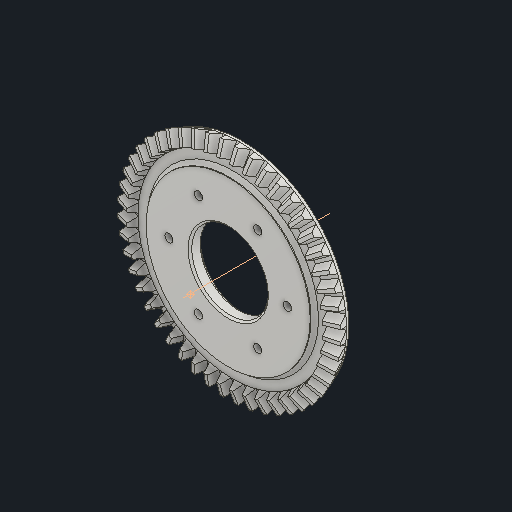
# Autodesk Inventor part: ENGRANAJE CÓNICO 1
Saved by Autodesk Inventor 2022 (Build 260153000, 153)
## iProperties
CustomPartVersion: 1
Created: 2021-09-21
Part Number: ENGRANAJE CÓNICO 1
Material: Steel, Mild
Document SubType Name: Modeling
Designer: Andres
Categories: <?xml version="1.0" encoding="UTF-16"?> <MemberInstance><Categories><FamilyTemplate><FamilyTemplateParameter ValueType="xs:double" Id="1" ObjectReferenceKey="da_z" ObjectType="kUserParameterObject"/><FamilyTemplateParameter ValueType="xs:double" Id="2" ObjectReferenceKey="da_b" ObjectType="kUserParameterObject"/><FamilyTemplateParameter ValueType="xs:double" Id="3" ObjectReferenceKey="da_beta" ObjectType="kUserParameterObject"/><FamilyTemplateParameter ValueType="xs:double" Id="4" ObjectReferenceKey="da_dae" ObjectType="kUserParameterObject"/><FamilyTemplateParameter ValueType="xs:double" Id="5" ObjectReferenceKey="da_ve" ObjectType="kUserParameterObject"/><FamilyTemplateParameter ValueType="xs:double" Id="6" ObjectReferenceKey="da_omega" ObjectType="kUserParameterObject"/><FamilyTemplateParameter ValueType="xs:string" Id="7" ObjectReferenceKey="EAIAABAAAAAAHwAAAAAAAIAAAAAAAAAA" ObjectType="83914240" SubObjectId="SurfaceGeometry"/></FamilyTemplate><ParamToTemplateMap><ParamToTemplate CategoryParameter="//CategoryParameter[@InternalName='046C89C9-8512-4d59-83FE-43B91F4F132A']" TemplateParameter="1"/><ParamToTemplate CategoryParameter="//CategoryParameter[@InternalName='2552DF32-E462-4b46-AEBF-C6C7768E72AC']" TemplateParameter="2"/><ParamToTemplate CategoryParameter="//CategoryParameter[@InternalName='C9EE641D-15FC-4fae-A226-E94C4372FDD7']" TemplateParameter="3"/><ParamToTemplate><ParamToTemplate CategoryParameter="//CategoryParameter[@InternalName='00B6519A-459B-49c7-AD84-2E56D39A5744']" ConstantValue="0.378492"/></ParamToTemplate><ParamToTemplate><ParamToTemplate CategoryParameter="//CategoryParameter[@InternalName='04B31F0E-C7A6-4894-AA32-9629BEFACF47']" ConstantValue="1.000000"/></ParamToTemplate><ParamToTemplate><ParamToTemplate CategoryParameter="//CategoryParameter[@InternalName='43CBEC2E-7847-49e7-A936-2F7889FCB2D9']" ConstantValue="0.200000"/></ParamToTemplate><ParamToTemplate><ParamToTemplate CategoryParameter="//CategoryParameter[@InternalName='B1EFC894-105D-4ebd-86BF-FA20ED196853']" ConstantValue="0.300000"/></ParamToTemplate><ParamToTemplate><ParamToTemplate CategoryParameter="//CategoryParameter[@InternalName='51175063-3D10-4879-93E8-6246FE8B403D']" ConstantValue="2060000000.000000"/></ParamToTemplate><ParamToTemplate><ParamToTemplate CategoryParameter="//CategoryParameter[@InternalName='A3A52E27-4454-46a9-B0BD-C932399B70AF']" ConstantValue="0.300000"/></ParamToTemplate><ParamToTemplate CategoryParameter="//CategoryParameter[@InternalName='2A200944-5A8C-41ca-B96E-8520D2E510F1']" TemplateParameter="4"/><ParamToTemplate><ParamToTemplate CategoryParameter="//CategoryParameter[@InternalName='1A637F62-92C8-44bc-B81F-10802510B579']" ConstantValue="10.734536"/></ParamToTemplate><ParamToTemplate CategoryParameter="//CategoryParameter[@InternalName='B52DD4BE-6863-48fb-BF58-89EF6F9EC65C']" TemplateParameter="5"/><ParamToTemplate><ParamToTemplate CategoryParameter="//CategoryParameter[@InternalName='3956BFF2-84D2-457d-93C2-9B0613DEBA67']" ConstantValue="1.799854"/></ParamToTemplate><ParamToTemplate CategoryParameter="//CategoryParameter[@InternalName='739CFA02-461B-4bf8-8049-181FCAD8B28F']" TemplateParameter="6"/><ParamToTemplate><ParamToTemplate CategoryParameter="//CategoryParameter[@InternalName='A27E999F-E2CE-4481-8A2A-EBF499C4C3C5']" ConstantValue="0.000000"/></ParamToTemplate><ParamToTemplate><ParamToTemplate CategoryParameter="//CategoryParameter[@InternalName='9E1B4470-B2D3-4ff1-B813-535BB4CDF51A']" ConstantValue="3160000.000000"/></ParamToTemplate><ParamToTemplate><ParamToTemplate CategoryParameter="//CategoryParameter[@InternalName='F8452263-BFF6-458c-9FB1-07C4B99E95CD']" ConstantValue="11400000.000000"/></ParamToTemplate><ParamToTemplate><ParamToTemplate CategoryParameter="//CategoryParameter[@InternalName='3E3BB259-FD49-497f-8171-6EBC954A3479']" ConstantValue="2.000000"/></ParamToTemplate><ParamToTemplate CategoryParameter="//CategoryParameter[@InternalName='27C3BAF2-7550-4e4b-AE2C-0DB134B7D9B7']" TemplateParameter="7"/></ParamToTemplateMap><Category DisplayName="Gear" InternalName="DC85795E-93AB-48d5-8EEE-5A27447B64BD" Mnemonic="Gear"><CategoryParameter DisplayName="z" InternalName="046C89C9-8512-4d59-83FE-43B91F4F132A" Mnemonic="z"/><CategoryParameter DisplayName="b" InternalName="2552DF32-E462-4b46-AEBF-C6C7768E72AC" Mnemonic="b"/><CategoryParameter DisplayName="||b|" InternalName="C9EE641D-15FC-4fae-A226-E94C4372FDD7" Mnemonic="beta"/><CategoryParameter DisplayName="x" InternalName="00B6519A-459B-49c7-AD84-2E56D39A5744" Mnemonic="x"/><CategoryParameter DisplayName="a*" InternalName="04B31F0E-C7A6-4894-AA32-9629BEFACF47" Mnemonic="a"/><CategoryParameter DisplayName="c*" InternalName="43CBEC2E-7847-49e7-A936-2F7889FCB2D9" Mnemonic="c"/><CategoryParameter DisplayName="r|.f|*" InternalName="B1EFC894-105D-4ebd-86BF-FA20ED196853" Mnemonic="rf"/><CategoryParameter DisplayName="E" InternalName="51175063-3D10-4879-93E8-6246FE8B403D" Mnemonic="E"/><CategoryParameter DisplayName="||m|" InternalName="A3A52E27-4454-46a9-B0BD-C932399B70AF" Mnemonic="mi"/><Category DisplayName="BevelGear" InternalName="0C98F69A-0C2B-4791-B2FE-7691BB227E77" Mnemonic="BevelGear"><CategoryParameter DisplayName="d|.ae|" InternalName="2A200944-5A8C-41ca-B96E-8520D2E510F1" Mnemonic="dae"/><CategoryParameter DisplayName="d|.ai|" InternalName="1A637F62-92C8-44bc-B81F-10802510B579" Mnemonic="dai"/><CategoryParameter DisplayName="A|.e|" InternalName="B52DD4BE-6863-48fb-BF58-89EF6F9EC65C" Mnemonic="ve"/><CategoryParameter DisplayName="A|.i|" InternalName="3956BFF2-84D2-457d-93C2-9B0613DEBA67" Mnemonic="vi"/><CategoryParameter DisplayName="||S|" InternalName="739CFA02-461B-4bf8-8049-181FCAD8B28F" Mnemonic="omega"/><CategoryParameter DisplayName="x|.t|" InternalName="A27E999F-E2CE-4481-8A2A-EBF499C4C3C5" Mnemonic="xt"/><CategoryParameter DisplayName="||s||.Flim|" InternalName="9E1B4470-B2D3-4ff1-B813-535BB4CDF51A" Mnemonic="sFlim"/><CategoryParameter DisplayName="||s||.Hlim|" InternalName="F8452263-BFF6-458c-9FB1-07C4B99E95CD" Mnemonic="sHlim"/><CategoryParameter DisplayName="type" InternalName="3E3BB259-FD49-497f-8171-6EBC954A3479" Mnemonic="type"/><CategoryParameter DisplayName="PitchDiameter" InternalName="27C3BAF2-7550-4e4b-AE2C-0DB134B7D9B7" Mnemonic="IDS_PITCHDIAM"/></Category></Category></Categories></MemberInstance>
Mass: 60.9118 g
Surface Area: 34.3074 cm^2
Volume: 7.7496 cm^3
Density: 7.86 g/cm^3
Appearance: Steel
Author: Andres
Autodesk Inventor part; units mm, degrees
ref_plane "Mesh Plane2" through (0, 0, 0) normal (0.9978589, 0.0654031, 0) x (0, 0, 1)
sketch "Teeth Body Sketch" plane through (0, 0, 0) normal (1, 0, 0) x (0, 1, 0)
  line L0 (0, 0) -> (59.2441, -25.6596) construction
  line L1 (59.2441, -25.6596) -> (61.2684, -20.5457)
  line L2 (61.2684, -20.5457) -> (0, 0) construction
  line L3 (60, -23.75) -> (0, 0) construction
  line L4 (51.8994, -22.4785) -> (53.6727, -17.9985)
  line L5 (59.2441, -25.6596) -> (51.8994, -22.4785)
  line L6 (61.2684, -20.5457) -> (53.6727, -17.9985)
  line L7 (0, -30.7915) -> (0, 5.1319) projected
  line L8 (0, -23.75) -> (61.2684, -23.75) construction
  dimension "d0" = 120
  dimension "d1" = 118.4882
  dimension "d2" = 122.5368
  dimension "d3" = 8
  dimension "d4" = 20.5457
  constraints: 16 end point, 4 point on line, 3 perpendicular, 2 collinear, 1 horizontal alignment, 1 vertical alignment
  measures "d0" diameter of L3.start L7
  measures "d1" diameter of L0.end L7
  measures "d2" diameter of L1.end L7
  measures "d3" distance between parallel lines of L1 L4
  measures "d4" vertical distance of L1.end L0.start
revolve "Teeth Body" add sketch "Teeth Body Sketch" angle 360 about axis through (0, 0, 0) along (0, 0, 1)
ref_plane "Tooth Plane" through (0, 60, -23.75) normal (0, -0.9298066, 0.3680485) x (1, 0, 0)
sketch "Start Sketch" plane through (0, 60, -23.75) normal (0, -0.9298066, 0.3680485) x (1, 0, 0)
  line L0 (0, -196.6479) -> (0, 38.7332) projected
  arc A0 (-0.741, -2.7138) -> (-3.7477, 5.0545) centre (-57.4116, -20.1822) ccw
  arc A1 (3.7477, 5.0545) -> (0.741, -2.7138) centre (57.4116, -20.1822) ccw
  line L1 (-0.741, -2.7138) -> (0.741, -2.7138)
  arc A2 (3.7477, 5.0545) -> (-3.7477, 5.0545) centre (0, -163.022) ccw
  dimension "d7" = 59.3018
  dimension "d8" = 57.4116
  dimension "d9" = 142.8398
  dimension "d57" = 168.1182
  dimension "d58" = 160.3082
  constraints: 6 point on circle, 3 centre point, 3 symmetric about line, 2 end point, 1 coincident, 1 perpendicular, 1 other
  measures "d7" radius of A0
  measures "d8" horizontal distance of point (0, -163.022) A0.centre
  measures "d9" vertical distance of point (0, -163.022) A0.centre
  measures "d57" radius of A2
  measures "d58" distance from line of A2.centre L1
sketch "End Sketch" plane through (0, 52.3059, -20.7044) normal (0, -0.9298066, 0.3680485) x (1, 0, 0)
  line L0 (0, -171.4306) -> (0, 33.7662) projected
  arc A0 (-0.646, -2.3658) -> (-3.2671, 4.4063) centre (-50.0494, -17.5941) ccw
  arc A1 (3.2671, 4.4063) -> (0.646, -2.3658) centre (50.0494, -17.5941) ccw
  line L1 (-0.646, -2.3658) -> (0.646, -2.3658)
  arc A2 (3.2671, 4.4063) -> (-3.2671, 4.4063) centre (0, -142.1168) ccw
  dimension "d12" = 51.6972
  dimension "d15" = 50.0494
  dimension "d16" = 124.5226
  dimension "d59" = 146.5595
  dimension "d60" = 139.751
  constraints: 6 point on circle, 3 centre point, 3 symmetric about line, 2 end point, 1 coincident, 1 other
  measures "d12" radius of A0
  measures "d15" horizontal distance of A0.centre point (0, -142.117)
  measures "d16" vertical distance of A0.centre point (0, -142.117)
  measures "d59" radius of A2
  measures "d60" distance from line of A2.centre L1
loft "Loft" cut profiles "Start Sketch", "End Sketch"
pattern_circular "Circular Pattern" count 48 over 360 about axis through (0, 0, 0) along (0, 0, 1) of "Loft"
ref_plane "End Plane" through (0, 52.3059, -20.7044) normal (0, -0.9298066, 0.3680485) x (1, 0, 0)
sketch3d "3D Sketch Right"
ref_plane "End Plane Right" through (-2.7978, 52.231, -20.7044) normal (0.0497347, -0.9284755, 0.3680485) x (0.9985684, 0.0534892, 0)
sketch "End Sketch Right" plane through (-2.7978, 52.231, -20.7044) normal (0.0497347, -0.9284755, 0.3680485) x (0.9985684, 0.0534892, 0)
  arc A0 (-0.646, -2.3658) -> (-3.2671, 4.4063) centre (-50.0494, -17.5941) ccw
  line L0 (0, -174.1855) -> (0, 36.5211) projected
  arc A1 (3.2671, 4.4063) -> (0.646, -2.3658) centre (50.0494, -17.5941) ccw
  line L1 (-0.646, -2.3658) -> (0.646, -2.3658)
  arc A2 (3.2671, 4.4063) -> (-3.2671, 4.4063) centre (0, -142.1168) ccw
  dimension "d70" = 50.0494
  dimension "d71" = 124.5226
  dimension "d72" = 51.6972
  dimension "d73" = 139.751
  dimension "d74" = 146.5595
  constraints: 6 point on circle, 3 centre point, 3 symmetric about line, 2 end point, 1 coincident, 1 perpendicular, 1 other
  measures "d70" horizontal distance of A2.centre A0.centre
  measures "d71" vertical distance of point (0, -142.117) A0.centre
  measures "d72" radius of A0
  measures "d73" distance from line of point (0, -142.117) L1
  measures "d74" radius of A2
feature "Loft Right" [suppressed]
pattern_circular "Circular Pattern Right" [suppressed]
sketch3d "3D Sketch Left"
ref_plane "End Plane Left" through (2.8193, 52.231, -20.7243) normal (-0.0501091, -0.928337, 0.3683469) x (0.9985464, -0.0538988, 0)
sketch "End Sketch Left" plane through (2.8193, 52.231, -20.7243) normal (-0.0501091, -0.928337, 0.3683469) x (0.9985464, -0.0538988, 0)
  line L0 (0, -174.3918) -> (0, 36.7636) projected
  arc A0 (-0.646, -2.3477) -> (-3.2671, 4.4244) centre (-50.0494, -17.576) ccw
  arc A1 (3.2671, 4.4244) -> (0.646, -2.3477) centre (50.0494, -17.576) ccw
  line L1 (-0.646, -2.3477) -> (0.646, -2.3477)
  ellipse E0 centre (0, -16.733) end of major axis (53.6727, -16.733) minor radius 19.7702 projected
  arc A2 (3.2671, 4.4244) -> (-3.2671, 4.4244) centre (0, -142.0987) ccw
  point P0 (0, -142.0987)
  dimension "d56" = 19.7702
  dimension "d30" = 51.6972
  dimension "d31" = 50.0494
  dimension "d32" = 124.5226
  dimension "d61" = 146.5595
  dimension "d62" = 139.751
  constraints: 6 point on circle, 3 centre point, 3 symmetric about line, 2 end point, 1 coincident, 2 other
  measures "d30" radius of A0
  measures "d31" horizontal distance of point (0, -142.099) A0.centre
  measures "d32" vertical distance of A0.centre point (0, -142.099)
  measures "d61" radius of A2
  measures "d62" distance from line of point (0, -142.099) L1
feature "Loft Left" [suppressed]
pattern_circular "Circular Pattern Left" [suppressed]
sketch "Body Sketch" plane through (0, 0, 0) normal (1, 0, 0) x (0, 1, 0)
  line L0 (0, -26.2958) -> (0, -21.8423) projected
  line L1 (59.2441, -25.6596) -> (51.8994, -22.4785) projected
  line L2 (51.8994, -22.4785) -> (0, -22.4785)
  line L3 (59.2441, -25.6596) -> (0, -25.6596)
  constraints: 4 end point, 2 perpendicular, 2 point on line
revolve "Fix Body" add sketch "Body Sketch" angle 360 about axis through (0, 0, 0) along (0, 0, 1)
sketch "Sketch6" plane through (0, 0, 0) normal (1, 0, 0) x (0, 1, 0)
  line L0 (60, -23.75) -> (0, 0) projected
  line L1 (0, -28.5) -> (0, 4.75) projected
surface revolve "Pitch Diameter" sketch "Sketch6" angle 360 about axis through (0, 0, 0) along (0, 0, 1) shown no curves L0
ref_plane "Work Plane6" through (-41, -41, -18) normal (0, 0, 1) x (1, 0, 0)
sketch "Sketch11" plane through (0, 0, -22.4785) normal (0, 0, 1) x (0.9978589, 0.0654031, 0)
  circle A0 centre (0, 0) radius 40 projected
  circle A1 centre (0, 0) radius 21
  dimension "d138" = 42
  constraints: 1 centre point, 1 coincident
  measures "d138" diameter of A1
extrude "Extrusion4" cut sketch "Sketch11" against normal through all contours A1
sketch "Sketch17" plane through (0, 0, -22.4785) normal (0, 0, 1) x (0.9978589, 0.0654031, 0)
  circle A0 centre (0, 0) radius 40 projected
  circle A1 centre (0, 0) radius 45
  circle A2 centre (0, 0) radius 21 projected
  point P0 (0, 0)
  dimension "d139" = 5
  constraints: 1 centre point
  measures "d139" radial gap between concentric circles of A0 A1
ref_plane "Work Plane9" through (-39, -39, -20) normal (0, 0, -1) x (0, 1, 0)
extrude "Extrusion9" add sketch "Sketch17" along normal up to surface (2.4785 mm away) contours A0 | A1
chamfer "Chamfer6" distance 2 angle 45 1 edges at (-44.9037, -2.9431, -22.4785)
chamfer "Chamfer7" distance 1 angle 45 1 edges at (-20.955, -1.3735, -20)
sketch "Sketch19" plane through (0, 0, -25.6596) normal (0, 0, -1) x (-0.9978589, 0.0654031, 0)
  circle A0 centre (0, 0) radius 21 projected
  arc A1 (4.8199, 59.0477) -> (2.9286, 59.1717) centre (0, 0) ccw projected
  arc A2 (2.9286, 59.1717) -> (-2.9286, 59.1717) centre (0, 0) ccw projected
  arc A3 (-2.9286, 59.1717) -> (-4.8199, 59.0477) centre (0, 0) ccw projected
  arc A4 (-4.8199, 59.0477) -> (-10.627, 58.2832) centre (0, 0) ccw projected
  arc A5 (-10.627, 58.2832) -> (-12.4859, 57.9134) centre (0, 0) ccw projected
  arc A6 (-12.4859, 57.9134) -> (-18.1436, 56.3975) centre (0, 0) ccw projected
  arc A7 (-18.1436, 56.3975) -> (-19.9383, 55.7883) centre (0, 0) ccw projected
  arc A8 (-19.9383, 55.7883) -> (-25.3497, 53.5468) centre (0, 0) ccw projected
  arc A9 (-25.3497, 53.5468) -> (-27.0496, 52.7085) centre (0, 0) ccw projected
  arc A10 (-27.0496, 52.7085) -> (-32.1221, 49.7799) centre (0, 0) ccw projected
  arc A11 (-32.1221, 49.7799) -> (-33.698, 48.7269) centre (0, 0) ccw projected
  arc A12 (-33.698, 48.7269) -> (-38.3449, 45.1612) centre (0, 0) ccw projected
  arc A13 (-38.3449, 45.1612) -> (-39.7698, 43.9116) centre (0, 0) ccw projected
  arc A14 (-39.7698, 43.9116) -> (-43.9116, 39.7698) centre (0, 0) ccw projected
  arc A15 (-43.9116, 39.7698) -> (-45.1612, 38.3449) centre (0, 0) ccw projected
  arc A16 (-45.1612, 38.3449) -> (-48.7269, 33.698) centre (0, 0) ccw projected
  arc A17 (-48.7269, 33.698) -> (-49.7799, 32.1221) centre (0, 0) ccw projected
  arc A18 (-49.7799, 32.1221) -> (-52.7085, 27.0496) centre (0, 0) ccw projected
  arc A19 (-52.7085, 27.0496) -> (-53.5468, 25.3497) centre (0, 0) ccw projected
  arc A20 (-53.5468, 25.3497) -> (-55.7883, 19.9383) centre (0, 0) ccw projected
  arc A21 (-55.7883, 19.9383) -> (-56.3975, 18.1436) centre (0, 0) ccw projected
  arc A22 (-56.3975, 18.1436) -> (-57.9134, 12.4859) centre (0, 0) ccw projected
  arc A23 (-57.9134, 12.4859) -> (-58.2832, 10.627) centre (0, 0) ccw projected
  arc A24 (-58.2832, 10.627) -> (-59.0477, 4.8199) centre (0, 0) ccw projected
  arc A25 (-59.0477, 4.8199) -> (-59.1717, 2.9286) centre (0, 0) ccw projected
  arc A26 (-59.1717, 2.9286) -> (-59.1717, -2.9286) centre (0, 0) ccw projected
  arc A27 (-59.1717, -2.9286) -> (-59.0477, -4.8199) centre (0, 0) ccw projected
  arc A28 (-59.0477, -4.8199) -> (-58.2832, -10.627) centre (0, 0) ccw projected
  arc A29 (-58.2832, -10.627) -> (-57.9134, -12.4859) centre (0, 0) ccw projected
  arc A30 (-57.9134, -12.4859) -> (-56.3975, -18.1436) centre (0, 0) ccw projected
  arc A31 (-56.3975, -18.1436) -> (-55.7883, -19.9383) centre (0, 0) ccw projected
  arc A32 (-55.7883, -19.9383) -> (-53.5468, -25.3497) centre (0, 0) ccw projected
  arc A33 (-53.5468, -25.3497) -> (-52.7085, -27.0496) centre (0, 0) ccw projected
  arc A34 (-52.7085, -27.0496) -> (-49.7799, -32.1221) centre (0, 0) ccw projected
  arc A35 (-49.7799, -32.1221) -> (-48.7269, -33.698) centre (0, 0) ccw projected
  arc A36 (-48.7269, -33.698) -> (-45.1612, -38.3449) centre (0, 0) ccw projected
  arc A37 (-45.1612, -38.3449) -> (-43.9116, -39.7698) centre (0, 0) ccw projected
  arc A38 (-43.9116, -39.7698) -> (-39.7698, -43.9116) centre (0, 0) ccw projected
  arc A39 (-39.7698, -43.9116) -> (-38.3449, -45.1612) centre (0, 0) ccw projected
  arc A40 (-38.3449, -45.1612) -> (-33.698, -48.7269) centre (0, 0) ccw projected
  arc A41 (-33.698, -48.7269) -> (-32.1221, -49.7799) centre (0, 0) ccw projected
  arc A42 (-32.1221, -49.7799) -> (-27.0496, -52.7085) centre (0, 0) ccw projected
  arc A43 (-27.0496, -52.7085) -> (-25.3497, -53.5468) centre (0, 0) ccw projected
  arc A44 (-25.3497, -53.5468) -> (-19.9383, -55.7883) centre (0, 0) ccw projected
  arc A45 (-19.9383, -55.7883) -> (-18.1436, -56.3975) centre (0, 0) ccw projected
  arc A46 (-18.1436, -56.3975) -> (-12.4859, -57.9134) centre (0, 0) ccw projected
  arc A47 (-12.4859, -57.9134) -> (-10.627, -58.2832) centre (0, 0) ccw projected
  arc A48 (-10.627, -58.2832) -> (-4.8199, -59.0477) centre (0, 0) ccw projected
  arc A49 (-4.8199, -59.0477) -> (-2.9286, -59.1717) centre (0, 0) ccw projected
  arc A50 (-2.9286, -59.1717) -> (2.9286, -59.1717) centre (0, 0) ccw projected
  arc A51 (2.9286, -59.1717) -> (4.8199, -59.0477) centre (0, 0) ccw projected
  arc A52 (4.8199, -59.0477) -> (10.627, -58.2832) centre (0, 0) ccw projected
  arc A53 (10.627, -58.2832) -> (12.4859, -57.9134) centre (0, 0) ccw projected
  arc A54 (12.4859, -57.9134) -> (18.1436, -56.3975) centre (0, 0) ccw projected
  arc A55 (18.1436, -56.3975) -> (19.9383, -55.7883) centre (0, 0) ccw projected
  arc A56 (19.9383, -55.7883) -> (25.3497, -53.5468) centre (0, 0) ccw projected
  arc A57 (25.3497, -53.5468) -> (27.0496, -52.7085) centre (0, 0) ccw projected
  arc A58 (27.0496, -52.7085) -> (32.1221, -49.7799) centre (0, 0) ccw projected
  arc A59 (32.1221, -49.7799) -> (33.698, -48.7269) centre (0, 0) ccw projected
  arc A60 (33.698, -48.7269) -> (38.3449, -45.1612) centre (0, 0) ccw projected
  arc A61 (38.3449, -45.1612) -> (39.7698, -43.9116) centre (0, 0) ccw projected
  arc A62 (39.7698, -43.9116) -> (43.9116, -39.7698) centre (0, 0) ccw projected
  arc A63 (43.9116, -39.7698) -> (45.1612, -38.3449) centre (0, 0) ccw projected
  arc A64 (45.1612, -38.3449) -> (48.7269, -33.698) centre (0, 0) ccw projected
  arc A65 (48.7269, -33.698) -> (49.7799, -32.1221) centre (0, 0) ccw projected
  arc A66 (49.7799, -32.1221) -> (52.7085, -27.0496) centre (0, 0) ccw projected
  arc A67 (52.7085, -27.0496) -> (53.5468, -25.3497) centre (0, 0) ccw projected
  arc A68 (53.5468, -25.3497) -> (55.7883, -19.9383) centre (0, 0) ccw projected
  arc A69 (55.7883, -19.9383) -> (56.3975, -18.1436) centre (0, 0) ccw projected
  arc A70 (56.3975, -18.1436) -> (57.9134, -12.4859) centre (0, 0) ccw projected
  arc A71 (57.9134, -12.4859) -> (58.2832, -10.627) centre (0, 0) ccw projected
  arc A72 (58.2832, -10.627) -> (59.0477, -4.8199) centre (0, 0) ccw projected
  arc A73 (59.0477, -4.8199) -> (59.1717, -2.9286) centre (0, 0) ccw projected
  arc A74 (59.1717, -2.9286) -> (59.1717, 2.9286) centre (0, 0) ccw projected
  arc A75 (59.1717, 2.9286) -> (59.0477, 4.8199) centre (0, 0) ccw projected
  arc A76 (59.0477, 4.8199) -> (58.2832, 10.627) centre (0, 0) ccw projected
  arc A77 (58.2832, 10.627) -> (57.9134, 12.4859) centre (0, 0) ccw projected
  arc A78 (57.9134, 12.4859) -> (56.3975, 18.1436) centre (0, 0) ccw projected
  arc A79 (56.3975, 18.1436) -> (55.7883, 19.9383) centre (0, 0) ccw projected
  arc A80 (55.7883, 19.9383) -> (53.5468, 25.3497) centre (0, 0) ccw projected
  arc A81 (53.5468, 25.3497) -> (52.7085, 27.0496) centre (0, 0) ccw projected
  arc A82 (52.7085, 27.0496) -> (49.7799, 32.1221) centre (0, 0) ccw projected
  arc A83 (49.7799, 32.1221) -> (48.7269, 33.698) centre (0, 0) ccw projected
  arc A84 (48.7269, 33.698) -> (45.1612, 38.3449) centre (0, 0) ccw projected
  arc A85 (45.1612, 38.3449) -> (43.9116, 39.7698) centre (0, 0) ccw projected
  arc A86 (43.9116, 39.7698) -> (39.7698, 43.9116) centre (0, 0) ccw projected
  arc A87 (39.7698, 43.9116) -> (38.3449, 45.1612) centre (0, 0) ccw projected
  arc A88 (38.3449, 45.1612) -> (33.698, 48.7269) centre (0, 0) ccw projected
  arc A89 (33.698, 48.7269) -> (32.1221, 49.7799) centre (0, 0) ccw projected
  arc A90 (32.1221, 49.7799) -> (27.0496, 52.7085) centre (0, 0) ccw projected
  arc A91 (27.0496, 52.7085) -> (25.3497, 53.5468) centre (0, 0) ccw projected
  arc A92 (25.3497, 53.5468) -> (19.9383, 55.7883) centre (0, 0) ccw projected
  arc A93 (19.9383, 55.7883) -> (18.1436, 56.3975) centre (0, 0) ccw projected
  arc A94 (18.1436, 56.3975) -> (12.4859, 57.9134) centre (0, 0) ccw projected
  arc A95 (12.4859, 57.9134) -> (10.627, 58.2832) centre (0, 0) ccw projected
  arc A96 (10.627, 58.2832) -> (4.8199, 59.0477) centre (0, 0) ccw projected
extrude "Extrusion10" add sketch "Sketch19" along normal blind 2
chamfer "Chamfer8" distance 2 angle 20 1 edges at (-0.9476, 59.2365, -27.6596) measured on face at (-0.9476, 59.2365, -27.1596)
sketch "Sketch20" plane through (0, 0, -27.6596) normal (0, 0, -1) x (-1, 0, 0)
  circle A0 centre (-16.25, 28.1458) radius 1.621 projected
  circle A1 centre (32.5, 0) radius 1.621 projected
  circle A2 centre (-16.25, -28.1458) radius 1.621 projected
  circle A3 centre (-32.5, 0) radius 1.621 projected
  circle A4 centre (16.25, -28.1458) radius 1.621 projected
  circle A5 centre (16.25, 28.1458) radius 1.621 projected
  circle A6 centre (0, 0) radius 39 projected
  circle A7 centre (0, 0) radius 22 projected
hole "Hole2" at (32.5, 0, -27.6596) at (16.25, -28.1458, -27.6596) at (-16.25, -28.1458, -27.6596) at (-32.5, 0, -27.6596) at (-16.25, 28.1458, -27.6596) at (16.25, 28.1458, -27.6596) direction (0, 0, 1) diameter 4.5 end through all counterbore diameter 8 counterbore depth 4.6 clearance for "Socket Head Cap Screw ISO 4762" size "M4" standard "ISO"
chamfer "Chamfer9" distance 2 angle 45 1 edges at (20.955, -1.3735, -27.6596)
equation "\"d0\" = da_de"
equation "\"d1\" = da_dfe"
equation "\"d2\" = da_dae"
equation "\"d3\" = da_b"
equation "\"d4\" = da_ve"
equation "\"d7\" = fd_rr"
equation "\"d8\" = fd_x"
equation "\"d9\" = fd_y"
equation "\"d57\" = 0.5 * fd_dva + 0.3 * da_he"
equation "\"d58\" = 0.5 * fd_dva - 1.12 * da_he"
equation "\"da_teethtype\" = 0"
equation "\"da_b\" = 8"
equation "\"da_de\" = 120"
equation "\"da_dae\" = 122.53676"
equation "\"da_dfe\" = 118.48823"
equation "\"da_le\" = 64.52955"
equation "\"da_omega\" = 90deg"
equation "\"da_beta\" = 0"
equation "\"da_delta\" = 68.40469deg"
equation "\"da_alpha\" = 20deg"
equation "\"da_he\" = 5.5"
equation "\"da_ve\" = 20.54567"
equation "\"da_zv\" = 130.417612"
equation "\"fd_loft\" = da_b + 0.05 * da_he"
equation "\"fd_x\" = fd_x1 + fd_x2"
equation "\"fd_y\" = fd_y1 - fd_y2"
equation "\"fd_dd\" = fd_dva - 0.8 * da_he"
equation "\"da_dvw\" = 327.93649"
equation "\"d11\" = fd_loft"
equation "\"da_dm\" = 112.56155"
equation "\"da_x\" = 0.378492"
equation "\"da_m\" = 2.5"
equation "\"d50\" = da_omega"
equation "\"fd_rr\" = 59.301777"
equation "\"fd_dva\" = 332.936487"
equation "\"fd_x1\" = 1.996786"
equation "\"fd_x2\" = 55.41484"
equation "\"fd_y1\" = 163.956085"
equation "\"fd_y2\" = 21.116257"
body "Solid1"
body "Srf1"
